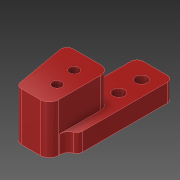
# Autodesk Inventor part: CH_01_0028_end_switch_mount_2
Saved by Autodesk Inventor 2022 (Build 260153000, 153)
## iProperties
Created: 2022-03-09
Part Number: CH_01_0028_end_switch_mount_2
Material: Generic
Document SubType Name: Modeling
Designer: Tomasz Krakowski
Density: 1 g/cm^3
Appearance: Czerwona
Author: Tomasz Krakowski
Autodesk Inventor part; units mm, degrees
ref_plane "YZ Plane" through (0, 0, 0) normal (1, 0, 0) x (0, 1, 0)
ref_plane "XZ Plane" through (0, 0, 0) normal (0, 1, 0) x (-1, 0, 0)
ref_plane "XY Plane" through (0, 0, 0) normal (0, 0, 1) x (1, 0, 0)
sketch "Sketch1" plane through (0, 0, 0) normal (0, 1, 0) x (-1, 0, 0)
  line L0 (0, 10) -> (0, -10)
  line L1 (0, 10) -> (8, 10)
  line L2 (8, 10) -> (11.5265, -10)
  line L3 (11.5265, -10) -> (0, -10)
  point P0 (0, 0)
  point P1 (0, 0)
  dimension "d0" = 100
  dimension "d1" = 20
  dimension "d2" = 8
  constraints: 8 end point, 1 coincident, 1 horizontal, 1 midpoint, 1 parallel, 1 vertical
  measures "d0" angle of L1 L2
  measures "d1" distance between parallel lines of L3 L1
  measures "d2" distance of L0.start L1.end
extrude "Extrusion1" add sketch "Sketch1" along normal blind 16
sketch "Sketch2" plane through (0, 16, 0) normal (0, 1, 0) x (1, 0, 0)
  line L0 (-1.6558, -2.7888) -> (-2.8714, 4.1049) construction
  line L1 (-2.2636, 0.658) -> (-9.6497, -0.6443) construction
  line L2 (-11.5265, 10) -> (-8, -10) construction
  point P0 (0, 0)
  dimension "d5" = 7
  dimension "d6" = 7.5
  dimension "d23" = 9.5
  constraints: 4 end point, 2 perpendicular, 1 midpoint, 1 point on line
  measures "d5" distance of L0.start L0.end
  measures "d6" distance of L1.end L1.start
  measures "d23" distance of L2.end L1.end
hole "Hole1" at (-1.6558, 16, 2.7888) at (-2.8714, 16, -4.1049) direction (0, -1, 0) diameter 3.1 depth 7.5
sketch "Sketch4" plane through (0, 0, 0) normal (0, -1, 0) x (1, 0, 0)
  line L0 (0, 4) -> (6, 4)
  line L1 (6, 4) -> (6, -28)
  line L2 (6, -28) -> (-6, -28)
  line L3 (-6, -28) -> (-6, -10)
  line L4 (0, -10) -> (-11.5265, -10) construction
  line L5 (0, 10) -> (0, -10) construction
  line L6 (0, 10) -> (0, -10) construction
  line L7 (0, 4) -> (0, -10)
  line L8 (0, -10) -> (-6, -10)
  point P0 (0, 0)
  dimension "d26" = 18
  dimension "d27" = 6
  dimension "d28" = 6
  dimension "d29" = 14
  constraints: 12 end point, 3 perpendicular, 1 collinear, 1 horizontal, 1 point on line, 1 vertical
  measures "d26" distance between parallel lines of L2 L4
  measures "d27" distance between parallel lines of L3 L5
  measures "d28" distance between parallel lines of L1 L5
  measures "d29" distance from line of L0 L4.start
extrude "Extrusion2" add sketch "Sketch4" against normal blind 6
sketch "Sketch5" plane through (0, 0, 0) normal (0, -1, 0) x (1, 0, 0)
  line L0 (1, -15) -> (1, -22.5) construction
  point P0 (0, 0)
  dimension "d34" = 7.5
  dimension "d43" = 15
  dimension "d44" = 1
  constraints: 2 end point, 1 vertical
  measures "d34" distance of L0.start L0.end
  measures "d43" vertical distance of L0.start point (0, 0)
  measures "d44" horizontal distance of point (0, 0) L0.start
hole "Hole3" at (1, 0, -15) at (1, 0, -22.5) direction (0, 1, 0) diameter 3.8 depth 10
fillet "Fillet2" radius 2 6 edges at (6, 3, 4) (-8, 8, 10) (6, 3, -28) (-6, 3, -28) (-11.5265, 8, -10) (-6, 3, -10)
sketch "Sketch7" plane through (0, 0, 0) normal (0, -1, 0) x (1, 0, 0)
  line L0 (0, 10) -> (0, 4) construction
  line L1 (0, 10) -> (3, 10)
  line L2 (3, 10) -> (3, -10)
  line L3 (3, -10) -> (0, -10)
  line L4 (0, -10) -> (0, 10)
  line L5 (-8, -10) -> (-9.143, -10) construction
  dimension "d45" = 3
  constraints: 8 end point, 2 parallel, 1 coincident, 1 horizontal, 1 perpendicular
  measures "d45" distance between parallel lines of L0 L2
extrude "Extrusion3" add sketch "Sketch7" against normal up to surface (16 mm away)
fillet "Fillet3" radius 3 3 edges at (3, 8, 10) (3, 11, -10) (3, 3, 4)
equation "\"d28\" = d27"
body "Solid1"
